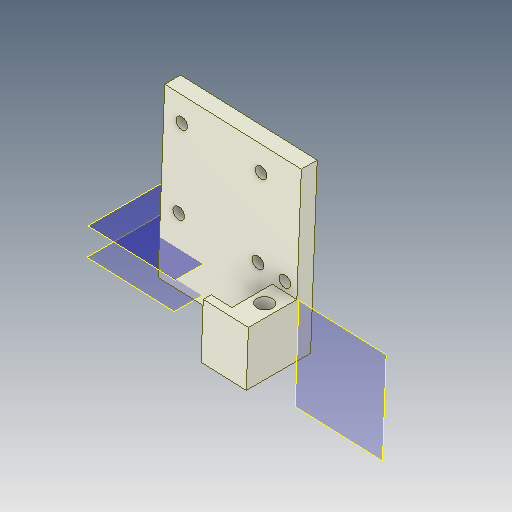
# Autodesk Inventor part: 30_cellSTORM_translation_y
Saved by Autodesk Inventor 2019.4 (Build 234330000, 330)
## iProperties
Created: 2021-07-02
Part Number: 30_cellSTORM_translation_y
Material: Generic
Document SubType Name: Modeling
Designer: diederichbenedict
Density: 1 g/cm^3
Appearance: Smooth - Ivory
Mass: 6.81065 g
Surface Area: 46.4405 cm^2
Volume: 6.81065 cm^3
Author: diederichbenedict
Autodesk Inventor part; units mm, degrees
ref_plane "YZ Plane" through (0, 0, 0) normal (1, 0, 0) x (0, 1, 0)
ref_plane "XZ Plane" through (0, 0, 0) normal (0, 1, 0) x (-1, 0, 0)
ref_plane "XY Plane" through (0, 0, 0) normal (0, 0, 1) x (1, 0, 0)
ref_plane "Work Plane3" through (68.5837, 137.6229, 5) normal (0, 0, -1) x (0.999249, -0.038749, 0)
sketch "Sketch3" plane through (68.5837, 137.6229, 5) normal (0, 0, -1) x (0.999249, -0.038749, 0)
  line L0 (-44.3, -40.7514) -> (-37.8, -40.7514) projected
  line L1 (-37.8, -8.3514) -> (-37.8, -40.7514) projected
  line L2 (-44.3, -8.3514) -> (-37.8, -8.3514) projected
  line L3 (-44.3, -8.3514) -> (-44.3, -40.7514) projected
  circle A0 centre (-41.4, -14.5514) radius 1.75 construction
  circle A1 centre (-41.4, -34.5514) radius 1.75 construction
  line L4 (-25, -40.7514) -> (-18.5, -40.7514) projected
  line L5 (-18.5, -8.3514) -> (-18.5, -40.7514) projected
  line L6 (-25, -8.3514) -> (-18.5, -8.3514) projected
  line L7 (-25, -8.3514) -> (-25, -40.7514) projected
  circle A2 centre (-21.4, -14.5514) radius 1.75 construction
  circle A3 centre (-21.4, -34.5514) radius 1.75 construction
  line L8 (-18.5, -40.7514) -> (-45.9422, -40.7514)
  line L9 (-45.9422, -40.7514) -> (-45.9422, -6.7531)
  line L10 (-45.9422, -6.7531) -> (-18.5, -6.7531)
  line L11 (-18.5, -6.7531) -> (-18.5, -40.7514)
  circle A4 centre (-41.4, -14.5514) radius 1.75 projected
  circle A5 centre (-41.4, -34.5514) radius 1.45
  circle A6 centre (-41.4, -14.5514) radius 1.45
  circle A7 centre (-21.4, -14.5514) radius 1.45
  circle A8 centre (-21.4, -34.5514) radius 1.45
  line L12 (-17.9, -8.3514) -> (-17.9, -40.7514) projected
  line L13 (-18.5, -40.7514) -> (-11.5, -40.7514)
  line L14 (-11.5, -40.7514) -> (-11.5, -8.3514)
  line L15 (-11.5, -8.3514) -> (-18.5, -8.3514)
  line L16 (-18.5, -8.3514) -> (-18.5, -40.7514)
  point P0 (-63.1994, 140.177)
  dimension "d12" = 2.9
  dimension "d13" = 2.9
  dimension "d14" = 2.9
  dimension "d15" = 2.9
  dimension "d16" = 7
  constraints: 16 end point, 4 centre point, 4 coincident, 4 parallel, 2 horizontal, 2 perpendicular
  measures "d12" diameter of A5
  measures "d13" diameter of A6
  measures "d14" diameter of A7
  measures "d15" diameter of A8
  measures "d16" distance of L15.end L14.end
extrude "Extrusion3" add sketch "Sketch3" along normal blind 4 contours L3 L2 L1 L0 | L8 L9 L10 L11 L6 L7 L1 L2 L3 | L7 L6 L5 L4 | L5 L15 L12 L13 | L12 L15 L14 L13 | A4
ref_plane "Work Plane4" through (22.9376, 146.1511, 1) normal (-0.038749, -0.999249, 0) x (0.999249, -0.038749, 0)
sketch "Sketch4" plane through (22.9376, 146.1511, 1) normal (-0.038749, -0.999249, 0) x (0.999249, -0.038749, 0)
  line L0 (27.4422, 4) -> (0, 4) projected
  line L1 (0, 4) -> (0, 0) projected
  line L2 (27.4422, 0) -> (0, 0) projected
  arc A0 (20.387, 12.6266) -> (19.8094, 12.1273) centre (20.8422, 11.5162) ccw construction
  arc A1 (19.616, 12.0055) -> (19.8094, 12.1273) centre (19.5942, 12.2545) ccw construction
  line L3 (19.616, 12.0055) -> (19.2704, 11.9753) construction
  arc A2 (19.2704, 11.9753) -> (19.0422, 11.7262) centre (19.2922, 11.7262) ccw construction
  line L4 (19.0422, 11.7262) -> (19.0422, 11.2738) construction
  arc A3 (19.0422, 11.2738) -> (19.2704, 11.0247) centre (19.2922, 11.2738) ccw construction
  line L5 (19.2704, 11.0247) -> (19.637, 10.9927) construction
  arc A4 (19.8267, 10.8768) -> (19.637, 10.9927) centre (19.6152, 10.7436) ccw construction
  arc A5 (19.8267, 10.8768) -> (20.387, 10.4059) centre (20.8422, 11.5162) ccw construction
  arc A6 (20.5422, 10.1746) -> (20.387, 10.4059) centre (20.2922, 10.1746) ccw construction
  line L6 (20.5422, 10.1746) -> (20.5422, 9.5) construction
  line L7 (20.5422, 9.5) -> (20.0422, 9) construction
  line L8 (20.0422, 9) -> (9.0422, 9) construction
  line L9 (9.0422, 9) -> (8.5422, 9.5) construction
  line L10 (8.5422, 9.5) -> (8.5422, 10.1746) construction
  arc A7 (8.6974, 10.4059) -> (8.5422, 10.1746) centre (8.7922, 10.1746) ccw construction
  arc A8 (8.6974, 10.4059) -> (9.2577, 10.8768) centre (8.2422, 11.5162) ccw construction
  arc A9 (9.4474, 10.9927) -> (9.2577, 10.8768) centre (9.4692, 10.7436) ccw construction
  line L11 (9.4474, 10.9927) -> (9.814, 11.0247) construction
  arc A10 (9.814, 11.0247) -> (10.0422, 11.2738) centre (9.7922, 11.2738) ccw construction
  line L12 (10.0422, 11.2738) -> (10.0422, 11.7262) construction
  arc A11 (10.0422, 11.7262) -> (9.814, 11.9753) centre (9.7922, 11.7262) ccw construction
  line L13 (9.814, 11.9753) -> (9.4684, 12.0055) construction
  arc A12 (9.275, 12.1273) -> (9.4684, 12.0055) centre (9.4902, 12.2545) ccw construction
  arc A13 (9.275, 12.1273) -> (8.6974, 12.6266) centre (8.2422, 11.5162) ccw construction
  arc A14 (8.5422, 12.8579) -> (8.6974, 12.6266) centre (8.7922, 12.8579) ccw construction
  line L14 (8.5422, 12.8579) -> (8.5422, 14) construction
  line L15 (8.5422, 14) -> (1.6422, 14) construction
  line L16 (1.6422, 14) -> (1.0422, 13.4) construction
  line L17 (1.0422, 13.4) -> (1.0422, 10) construction
  arc A15 (1.0422, 9.2) -> (1.0422, 10) centre (0.7422, 9.6) ccw construction
  line L18 (1.0422, 9.2) -> (1.0422, 4.6) construction
  line L19 (1.0422, 4.6) -> (1.6422, 4) construction
  line L20 (1.6422, 4) -> (8.1422, 4) construction
  line L21 (8.1422, 4) -> (8.5422, 4.4) construction
  line L22 (8.5422, 4.4) -> (20.5422, 4.4) construction
  line L23 (20.5422, 4.4) -> (20.9422, 4) construction
  line L24 (20.9422, 4) -> (27.4422, 4) construction
  line L25 (27.4422, 4) -> (28.0422, 4.6) construction
  line L26 (28.0422, 4.6) -> (28.0422, 13.4) construction
  line L27 (28.0422, 13.4) -> (27.4422, 14) construction
  line L28 (27.4422, 14) -> (20.5422, 14) construction
  line L29 (20.5422, 14) -> (20.5422, 12.8579) construction
  arc A16 (20.387, 12.6266) -> (20.5422, 12.8579) centre (20.2922, 12.8579) ccw construction
  line L30 (0, 4) -> (34.4422, 4) projected
  line L31 (34.4422, 4) -> (28.2422, 4)
  line L32 (28.2422, 4) -> (28.2422, 16.2)
  line L33 (28.2422, 16.2) -> (34.4422, 16.2)
  line L34 (34.4422, 16.2) -> (34.4422, 4)
  line L35 (28.2422, 16.2) -> (23.0467, 16.2)
  line L36 (23.0467, 16.2) -> (23.0467, 14.2)
  line L37 (23.0467, 14.2) -> (28.2422, 14.2)
  line L38 (28.2422, 14.2) -> (28.2422, 16.2)
  circle A17 centre (31.3422, 9) radius 2
  line L39 (27.4422, 4) -> (27.4422, 0) projected
  line L40 (27.4422, 0) -> (34.4422, 0)
  line L41 (34.4422, 0) -> (34.4422, 4)
  line L42 (34.4422, 4) -> (27.4422, 4)
  line L43 (27.4422, 4) -> (27.4422, 0)
  point P0 (-17.2572, -1)
  dimension "d17" = 0.2
  dimension "d18" = 0.2
  dimension "d19" = 2
  dimension "d20" = 4
  constraints: 24 end point, 6 parallel, 3 horizontal, 3 perpendicular, 1 centre point
  measures "d17" distance between parallel lines of L32 L26
  measures "d18" distance between parallel lines of L28 L37
  measures "d19" distance between parallel lines of L37 L35
  measures "d20" diameter of A17
extrude "Extrusion4" add sketch "Sketch4" against normal blind 5
ref_plane "Work Plane5" through (22.9376, 146.1511, 1) normal (-0.038749, -0.999249, 0) x (0.999249, -0.038749, 0)
sketch "Sketch6" plane through (22.9376, 146.1511, 1) normal (-0.038749, -0.999249, 0) x (0.999249, -0.038749, 0)
  line L0 (27.4422, 4) -> (0, 4) projected
  line L1 (0, 4) -> (0, 0) projected
  line L2 (27.4422, 0) -> (0, 0) projected
  line L3 (27.4422, 4) -> (27.4422, 0) projected
  line L4 (28.2422, 14.2) -> (23.0467, 14.2) projected
  line L5 (23.0467, 14.2) -> (28.2422, 14.2)
  line L6 (28.2422, 14.2) -> (28.2422, 4)
  line L7 (28.2422, 4) -> (23.0467, 4)
  line L8 (23.0467, 4) -> (23.0467, 14.2)
  line L9 (27.4422, 4) -> (28.2422, 4) projected
  line L10 (27.4422, 4) -> (27.4422, 0) projected
  line L11 (34.4422, 0) -> (27.4422, 0) projected
  line L12 (34.4422, 4) -> (34.4422, 0) projected
  line L13 (28.2422, 4) -> (34.4422, 4) projected
  circle A0 centre (31.3422, 9) radius 2 projected
  line L14 (34.4422, 16.2) -> (23.0467, 16.2) projected
  line L15 (23.0467, 16.2) -> (23.0467, 14.2) projected
  line L16 (23.0467, 14.2) -> (28.2422, 14.2) projected
  line L17 (28.2422, 4) -> (28.2422, 14.2) projected
  line L18 (34.4422, 16.2) -> (34.4422, 0) projected
  line L19 (28.2422, 4) -> (0, 4) projected
  line L20 (0, 4) -> (0, 0) projected
  line L21 (0, 0) -> (34.4422, 0) projected
  point P0 (-17.2572, -1)
  constraints: 8 end point, 2 parallel, 1 horizontal, 1 perpendicular
extrude "Extrusion6" add sketch "Sketch6" along normal blind 7 contours L3 L2 L1 L0 | L7 L13 L12 L11 L3 | L6 L4 L15 L14 L18 L13
ref_plane "Work Plane6" through (22.6664, 139.1564, 1) normal (-0.038749, -0.999249, 0) x (0.999249, -0.038749, 0)
sketch "Sketch7" plane through (22.6664, 139.1564, 1) normal (-0.038749, -0.999249, 0) x (0.999249, -0.038749, 0)
  circle A0 centre (31.3422, 9) radius 2 projected
  line L0 (28.2422, 4) -> (0, 4) projected
  line L1 (0, 4) -> (0, 0) projected
  line L2 (0, 0) -> (34.4422, 0) projected
  line L3 (23.0467, 14.2) -> (23.0467, 16.2) projected
  line L4 (28.2422, 4) -> (34.4422, 4) projected
  line L5 (23.0467, 14.2) -> (28.2422, 14.2)
  line L6 (28.2422, 14.2) -> (28.2422, 4)
  line L7 (28.2422, 4) -> (23.0467, 4)
  line L8 (23.0467, 4) -> (23.0467, 14.2)
  line L9 (34.4422, 0) -> (34.4422, 16.2) projected
  line L10 (34.4422, 16.2) -> (23.0467, 16.2) projected
  line L11 (23.0467, 16.2) -> (23.0467, 14.2) projected
  line L12 (23.0467, 14.2) -> (28.2422, 14.2) projected
  line L13 (28.2422, 14.2) -> (28.2422, 4) projected
  point P0 (-17.2572, -1)
  constraints: 8 end point, 2 parallel, 1 horizontal, 1 perpendicular
extrude "Extrusion7" add sketch "Sketch7" along normal blind 2
sketch "Sketch5" plane through (22.5889, 137.1579, 1) normal (0.038749, 0.999249, 0) x (0.999249, -0.038749, 0)
  circle A0 centre (31.3422, -9) radius 2 projected
  line L0 (28.5922, -10.5877) -> (28.5922, -7.4123)
  line L1 (28.5922, -7.4123) -> (31.3422, -5.8246)
  line L2 (31.3422, -5.8246) -> (34.0922, -7.4123)
  line L3 (34.0922, -7.4123) -> (34.0922, -10.5877)
  line L4 (34.0922, -10.5877) -> (31.3422, -12.1754)
  line L5 (31.3422, -12.1754) -> (28.5922, -10.5877)
  point P0 (-17.2572, 1)
  point P1 (31.3422, -9)
  dimension "d23" = 0
  dimension "d24" = 5.5
  constraints: 12 end point, 1 coincident, 13 other
  measures "d23" horizontal distance of L0.start L0.end
  measures "d24" distance between parallel lines of L0 L3
extrude "Extrusion5" cut sketch "Sketch5" along normal blind 4
sketch "Sketch8" plane through (68.5837, 137.6229, 1) normal (0, 0, -1) x (-0.999249, 0.038749, 0)
  line L0 (22.8955, 11.7531) -> (11.5, 11.7531) projected
  line L1 (12.6, 1.7531) -> (16.6, 1.7531) projected
  circle A0 centre (14.6, 14.0688) radius 1.45
  point P0 (63.1994, -140.177)
  dimension "d31" = 2.9
  constraints: 1 centre point
  measures "d31" diameter of A0
extrude "Extrusion8" cut sketch "Sketch8" against normal up to surface
sketch "Sketch9" plane through (22.5889, 137.1579, 1) normal (-0.038749, -0.999249, 0) x (0.999249, -0.038749, 0)
  circle A0 centre (15.7007, 11.4189) radius 1.45 projected
  point P0 (-17.2572, -1)
extrude "Extrusion9" cut sketch "Sketch9" against normal blind 5
equation "\"d32\" = d31"
body "Solid2"
